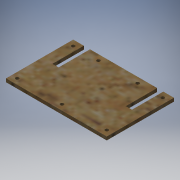
# Autodesk Inventor part: bottom
Saved by Autodesk Inventor 2018 (Build 220112000, 112)
## iProperties
Created: 2019-06-17
Part Number: bottom
Material: Generic
Document SubType Name: Modeling
Designer: ZEUSLAP
Density: 1 g/cm^3
Appearance: Default
Author: ZEUSLAP
Autodesk Inventor part; units mm, degrees
ref_plane "YZ Plane" through (0, 0, 0) normal (1, 0, 0) x (0, 1, 0)
ref_plane "XZ Plane" through (0, 0, 0) normal (0, 1, 0) x (-1, 0, 0)
ref_plane "XY Plane" through (0, 0, 0) normal (0, 0, 1) x (1, 0, 0)
sketch "Sketch1" plane through (0, 0, 0) normal (0, 0, 1) x (1, 0, 0)
  line L0 (-70, 40) -> (70, 40) construction
  line L1 (70, 40) -> (70, -40) construction
  line L2 (70, -40) -> (-70, -40) construction
  line L3 (-70, -40) -> (-70, 40) construction
  line L4 (90, 60) -> (-90, 60)
  line L5 (-90, 60) -> (-90, -60)
  line L6 (-90, -60) -> (90, -60)
  line L7 (90, -60) -> (90, 60)
  circle A0 centre (80, 50) radius 3
  circle A1 centre (-80, 50) radius 3
  circle A2 centre (-80, -50) radius 3
  circle A3 centre (0, -50) radius 3
  circle A4 centre (80, -50) radius 3
  line L8 (-90, 0) -> (90, 0) construction
  line L9 (0, 60) -> (0, -60) construction
  line L10 (-71, 60) -> (-71, 4)
  line L11 (-71, 4) -> (-60, 4)
  line L12 (-60, 4) -> (-60, 60)
  line L13 (71, 60) -> (71, 4)
  line L14 (71, 4) -> (60, 4)
  line L15 (60, 4) -> (60, 60)
  circle A5 centre (-35, 50) radius 3
  circle A6 centre (35, 50) radius 3
  point P0 (0, 0)
  point P1 (0, 40)
  point P2 (70, 0)
  point P3 (-70, 0)
  point P4 (0, 0)
  dimension "d0" = 140
  dimension "d1" = 80
  dimension "d2" = 20
  dimension "d7" = 6
  dimension "d8" = 10
  dimension "d9" = 10
  dimension "d17" = 56
  dimension "d18" = 11
  dimension "d19" = 1
  dimension "d20" = 10
  dimension "d21" = 35
  constraints: 32 end point, 8 midpoint, 7 centre point, 6 perpendicular, 5 equal radius, 4 parallel, 4 point on line, 2 vertical, 1 horizontal, 1 horizontal alignment, 1 vertical alignment, 11 other
  measures "d0" distance of L1.end L2.end
  measures "d1" distance of L0.end L1.end
  measures "d2" distance between parallel lines of L0 L4
  measures "d7" diameter of A1
  measures "d8" distance from line of L5 A1.centre
  measures "d9" distance from line of L4 A1.centre
  measures "d17" distance of L10.start L10.end
  measures "d18" distance of L10.end L11.end
  measures "d19" distance between parallel lines of L10 L3
  measures "d20" distance from line of L4 A5.centre
  measures "d21" distance from line of L9 A5.centre
extrude "Extrusion3" add sketch "Sketch1" along normal blind 6 contours L7 L6 L5 L4 L10 L11 L12 L15 L14 L13
body "Solid3"
